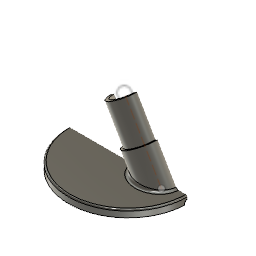
al-base-plate (Autodesk Fusion 360 design; units mm, degrees)
Autodesk Fusion 360 part; units mm, degrees
sketch "Skizze1" plane through (0, 0, 0) normal (0, 0, 1) x (1, 0, 0)
  circle A0 centre (0, 0) radius 80
extrude "Extrusion1" add sketch "Skizze1" along normal blind 10 makes body 1
fillet "Abrundung1" radius 2 1 edges at (-74.5862, -28.9292, 10) on bodies 1
sketch "Skizze2" plane through (0, 0, 0) normal (0, 1, 0) x (1, 0, 0)
  line L0 (45, 0) -> (-5, -86.6025) construction
ref_plane "Arbeitsebene1" through (-5, 0, 86.6025) normal (-0.5, 0, 0.866025) x (0, -1, 0)
sketch "Skizze3" plane through (-5, 0, 86.6025) normal (-0.5, 0, 0.866025) x (0, -1, 0)
  circle A0 centre (0, 0) radius 23
  circle A1 centre (0, 0) radius 20
extrude "Extrusion5" add sketch "Skizze3" against normal blind 110 separate body contours A0 | A1 makes body 2
combine "Kombinieren1" operation add target body 1 tool bodies 2
extrude "Extrusion6" cut sketch "Skizze3" against normal blind 50 bodies 1
fillet "Abrundung2" radius 4 3 edges at (65.7846, 0, 10) (-74.5862, -28.9292, 8) (-72.7215, 28.206, 10) on bodies 1
sketch "Skizze4" plane through (-5, 0, 86.6025) normal (-0.5, 0, 0.866025) x (0, -1, 0)
  circle A0 centre (0, 0) radius 15.75
extrude "Extrusion7" cut sketch "Skizze4" against normal blind 110 bodies 1
sketch "Skizze5" plane through (0, 0, 0) normal (0, 0, 1) x (1, 0, 0)
  circle A0 centre (0, 0) radius 160
extrude "Extrusion8" cut sketch "Skizze5" against normal blind 110 bodies 1
sketch "Skizze6" plane through (0, 0, 0) normal (0, 0, 1) x (1, 0, 0)
  line L0 (45, 0) -> (85, 0)
ref_plane "Arbeitsebene2" through (45, 0, 0) normal (1, 0, 0) x (0, 1, 0)
sketch "Skizze7" plane through (45, 0, 0) normal (1, 0, 0) x (0, 1, 0)
  line L0 (-4, 0) -> (-4, 1.7)
  line L1 (-4, 1.7) -> (-3.2, 3.3)
  line L2 (-3.2, 3.3) -> (-1, 5.5)
  line L3 (-1, 5.5) -> (1, 5.5)
  line L4 (1, 5.5) -> (3.2, 3.3)
  line L5 (3.2, 3.3) -> (4, 1.7)
  line L6 (4, 1.7) -> (4, 0)
  line L7 (4, 0) -> (-4, 0)
sweep "Sweeping1" cut profiles "Skizze7" path "Skizze6" along L0 section 1 bodies 1
sketch "Skizze8" plane through (0, 0, 0) normal (0, 0, 1) x (1, 0, 0)
  circle A0 centre (0, 0) radius 72.5
extrude "Extrusion9" cut sketch "Skizze8" along normal blind 3 bodies 1
sketch "Skizze9" plane through (0, 0, 0) normal (0, 0, 1) x (1, 0, 0)
  line L0 (72.2241, -6.3188) -> (73.7184, -6.4495)
  line L1 (73.7184, -6.4495) -> (69.5373, 25.3095)
  line L2 (69.5373, 25.3095) -> (68.1277, 24.7965)
  line L3 (68.1277, 24.7965) -> (72.2241, -6.3188)
  line L4 (6.3188, 72.2241) -> (6.4495, 73.7184)
  line L5 (6.4495, 73.7184) -> (-25.3095, 69.5373)
  line L6 (-25.3095, 69.5373) -> (-24.7965, 68.1277)
  line L7 (-24.7965, 68.1277) -> (6.3188, 72.2241)
  line L8 (-72.2241, 6.3188) -> (-73.7184, 6.4495)
  line L9 (-73.7184, 6.4495) -> (-69.5373, -25.3095)
  line L10 (-69.5373, -25.3095) -> (-68.1277, -24.7965)
  line L11 (-68.1277, -24.7965) -> (-72.2241, 6.3188)
  line L12 (-6.3188, -72.2241) -> (-6.4495, -73.7184)
  line L13 (-6.4495, -73.7184) -> (25.3095, -69.5373)
  line L14 (25.3095, -69.5373) -> (24.7965, -68.1277)
  line L15 (24.7965, -68.1277) -> (-6.3188, -72.2241)
extrude "Extrusion10" cut sketch "Skizze9" along normal blind 1.2 from surface at 1.8 bodies 1
sketch "Skizze10" plane through (0, 0, 0) normal (0, 0, 1) x (1, 0, 0)
  circle A0 centre (0, 0) radius 72.3
  line L0 (71.1263, -4.9736) -> (73.6202, -5.148)
  line L1 (73.6202, -5.148) -> (73.6202, 5.148)
  line L2 (73.6202, 5.148) -> (71.1263, 4.9736)
  line L3 (71.1263, 4.9736) -> (71.1263, -4.9736)
  line L4 (4.9736, 71.1263) -> (5.148, 73.6202)
  line L5 (5.148, 73.6202) -> (-5.148, 73.6202)
  line L6 (-5.148, 73.6202) -> (-4.9736, 71.1263)
  line L7 (-4.9736, 71.1263) -> (4.9736, 71.1263)
  line L8 (-71.1263, 4.9736) -> (-73.6202, 5.148)
  line L9 (-73.6202, 5.148) -> (-73.6202, -5.148)
  line L10 (-73.6202, -5.148) -> (-71.1263, -4.9736)
  line L11 (-71.1263, -4.9736) -> (-71.1263, 4.9736)
  line L12 (-4.9736, -71.1263) -> (-5.148, -73.6202)
  line L13 (-5.148, -73.6202) -> (5.148, -73.6202)
  line L14 (5.148, -73.6202) -> (4.9736, -71.1263)
  line L15 (4.9736, -71.1263) -> (-4.9736, -71.1263)
extrude "Extrusion11" add sketch "Skizze10" along normal blind 3 separate body makes body 3
sketch "Skizze11" plane through (0, 0, 0) normal (0, 0, 1) x (1, 0, 0)
  circle A0 centre (0, 39.875) radius 9
  circle A1 centre (0, -39.875) radius 9
extrude "Extrusion12" cut sketch "Skizze11" along normal blind 1.5 bodies 3
chamfer "Fase1" distance 0.5 angle 45 1 edges at (73.6202, 0, 3) on bodies 3
equation "base_plate_diameter = 160 mm" comment "Durchmesser der runden Basis-Platte"
equation "base_plate_height = 10 mm" comment "Höhe der runden Basis-Platte"
equation "base_plate_rounding = 2 mm" comment "Abrundung der oberen Basis-Platte-Kante (Kreis)"
equation "leg_outer_diameter = 46 mm" comment "Aussendurchmesser der Röhre"
equation "ring_inner_diameter = 40 mm" comment "Aussendurchmesser des oberen Röhrensegments (Stufenabsatz)"
equation "ring_extrude_depth = 50 mm" comment "Länge des oberen (dünnen) Röhrensegments / Stufenabsatz"
equation "hole_inner_diameter = 31.5 mm" comment "Innendurchmesser der Röhre (Loch)"
equation "leg_length = 100 mm" comment "Laenge der Röhre"
equation "leg_angle = 120 deg" comment "Winkel des Beines zur XY-Ebene (Innenwinkel an der Platte)"
equation "leg_offset = 45 mm" comment "Abstand des Bein-Fußpunktes vom Plattenmittelpunkt"
equation "leg_plate_rounding = 4 mm" comment "Abrundung der Kante: Bein und Platte (wird bei Solver-Problemen automatisch verkleinert)"
equation "cable_channel_width = 8 mm" comment "Breite des unterseitigen Kabelkanals"
equation "cable_channel_depth = 5.5 mm" comment "Gesamttiefe des unterseitigen Kabelkanals"
equation "cable_channel_vertical_height = 2.5 mm" comment "Höhe des senkrechten Wand-Abschnitts des Kabelkanals"
equation "cable_channel_edge_chamfer = 0.8 mm" comment "Abfasung der Kante zwischen senkrechter Wand und 45°-Dach im Kabelkanal"
equation "cover_plate_diameter = 145 mm" comment "Durchmesser der unterseitigen Abdeckplatte (Vertiefung)"
equation "cover_plate_thickness = 3 mm" comment "Dicke der unterseitigen Abdeckplatte"
equation "finger_grip_diameter = 18 mm" comment "Durchmesser der Finger-Vertiefungen zum Drehen der Abdeckplatte"
equation "finger_grip_depth = 1.5 mm" comment "Tiefe der Finger-Vertiefungen an der Unterseite der Abdeckplatte"
equation "clamp_recess_width = 22 mm" comment "Breite der Klemmsteg-Vertiefung quer zum Kanal"
equation "clamp_recess_length = 12 mm" comment "Länge der Klemmsteg-Vertiefung entlang des Kanals"
equation "clamp_recess_depth = 2.5 mm" comment "Tiefe der Klemmsteg-Vertiefung an der Unterseite"
equation "strain_relief_screw_diameter = 2.6 mm" comment "Bohrungsdurchmesser für M3-Zugsicherungsschellen"
equation "strain_relief_screw_depth = 6 mm" comment "Bohrungstiefe für M3-Zugsicherungsschellen"
equation "d25 = base_plate_height"
equation "d28 = base_plate_rounding"
equation "d36 = -( leg_length + base_plate_height )"
equation "d38 = -ring_extrude_depth"
equation "d41 = leg_plate_rounding"
equation "d42 = -leg_length - base_plate_height"
equation "d44 = -( leg_length + base_plate_height )"
equation "d53 = cover_plate_thickness"
equation "d58 = cover_plate_thickness"
equation "d60 = finger_grip_depth"
